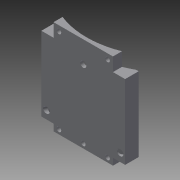
# Autodesk Inventor part: gauntlet mount
Saved by Autodesk Inventor 2014 SP1 (Build 180222100, 222)
## iProperties
Created: 2014-07-12
Part Number: gauntlet mount
Material: Generic
Document SubType Name: Modeling
Designer: Nick
Density: 1 g/cm^3
Appearance: Default
Author: Nick
Autodesk Inventor part; units mm, degrees
sketch "Sketch1" plane through (0, 0, 0) normal (0, 0, 1) x (1, 0, 0)
  line L0 (5, -2.4742) -> (53, -2.4742) construction
  line L1 (-26.0057, 3.6603) -> (-26.0057, -3.8397)
  arc A0 (0, 0) -> (58, 0) centre (29, 52.3167) ccw
  line L2 (60, -10) -> (-2, -10)
  line L3 (58, 0) -> (60, 0)
  line L4 (60, 0) -> (60, -10)
  line L5 (0, 0) -> (-2, 0)
  line L6 (-2, 0) -> (-2, -10)
  dimension "d0" = 48
  dimension "d1" = 7.5
  dimension "d2" = 58
  dimension "d16" = 2
  dimension "d17" = 2
  dimension "d18" = 10
  constraints: 14 end point, 4 perpendicular, 4 point on circle, 1 centre point, 1 horizontal, 1 parallel, 1 other
  measures "d0" distance of L0.start L0.end
  measures "d1" distance of L1.start L1.end
  measures "d2" distance of L5.start L3.start
  measures "d16" distance of L3.start L3.end
  measures "d17" distance of L5.start L5.end
  measures "d18" distance of L3.end L2.start
extrude "Extrusion1" add sketch "Sketch1" along normal blind 12
sketch3d "3D Sketch1"
ref_plane "Work Plane1" through (5, -2.4742, 6) normal (0.401226, 0.9159791, 0) x (-0.9159791, 0.401226, 0)
ref_plane "Work Plane2" through (53, -2.4742, 6) normal (-0.401226, 0.9159791, 0) x (-0.9159791, -0.401226, 0)
sketch "Sketch2" plane through (53, -2.4742, 6) normal (-0.401226, 0.9159791, 0) x (-0.9159791, -0.401226, 0)
  circle A0 centre (0, 0) radius 2.25
  point P0 (47.5542, -6)
  dimension "d9" = 4.5
  constraints: 1 centre point
  measures "d9" diameter of A0
extrude "Extrusion2" cut sketch "Sketch2" along normal mid plane 30
sketch "Sketch3" plane through (5, -2.4742, 6) normal (0.401226, 0.9159791, 0) x (-0.9159791, 0.401226, 0)
  circle A0 centre (0, 0) radius 2.25
  point P0 (5.5726, -6)
  dimension "d12" = 4.5
  constraints: 1 centre point
  measures "d12" diameter of A0
extrude "Extrusion3" cut sketch "Sketch3" along normal mid plane 30
thicken "Thicken1" operation add thickness 43 both sides no extend neighbours yes toward (0, 0, 1) faces at (29, -9.1667, 12)
sketch "Sketch4" plane through (-2, -10, 0) normal (0, -1, 0) x (1, 0, 0)
  line L0 (62, 0) -> (0, 0) projected
  line L1 (0, 55) -> (62, 55) projected
  circle A0 centre (31, 49) radius 2.25
  point P0 (2, 0)
  point P1 (31, 55)
  dimension "d21" = 4.5
  dimension "d22" = 49
  constraints: 1 centre point, 1 midpoint, 1 vertical alignment
  measures "d21" diameter of A0
  measures "d22" distance from line of L0 A0.centre
extrude "Extrusion4" cut sketch "Sketch4" against normal blind 15
sketch "Sketch5" plane through (0, 0, 0) normal (0, 0, -1) x (-1, 0, 0)
  line L0 (-58.7529, -10) -> (-55.044, -1.5326) projected
  line L1 (-53.8402, -10) -> (-50.9221, -3.3381) projected
  line L2 (0.7529, -10) -> (-2.956, -1.5326) projected
  line L3 (-4.1598, -10) -> (-7.0779, -3.3381) projected
  line L4 (-57.6988, -3.6449) -> (-59.063, -6.7592)
  line L5 (-59.063, -6.7592) -> (-52.2847, -9.7283)
  line L6 (-52.2847, -9.7283) -> (-50.9206, -6.614)
  line L7 (-50.9206, -6.614) -> (-57.6988, -3.6449)
  dimension "d25" = 7.4
  dimension "d26" = 3.4
  dimension "d27" = 3
  constraints: 8 end point, 3 parallel, 1 perpendicular
  measures "d25" distance of L4.end L5.end
  measures "d26" distance of L5.end L6.end
  measures "d27" distance from line of L7 L1.end
extrude "Extrusion5" cut sketch "Sketch5" against normal blind 10.5
ref_plane "Work Plane3" through (29, -10, 0) normal (1, 0, 0) x (0, 0, -1)
mirror "Mirror1" about plane through (29, -10, 0) normal (1, 0, 0) of "Extrusion5"
sketch "Sketch6" plane through (-2, -10, 0) normal (0, -1, 0) x (1, 0, 0)
  line L0 (62, 0) -> (0, 0) projected
  circle A0 centre (31, -1.75) radius 1.7
  circle A1 centre (49, -1.75) radius 1.7
  circle A2 centre (13, -1.75) radius 1.7
  line L1 (9, -5) -> (53, -5)
  line L2 (53, -5) -> (53, 0)
  line L3 (53, 0) -> (9, 0)
  line L4 (9, 0) -> (9, -5)
  line L5 (0, 55) -> (62, 55) projected
  line L6 (9, 55) -> (53, 55)
  line L7 (53, 55) -> (53, 65)
  line L8 (53, 65) -> (9, 65)
  line L9 (9, 65) -> (9, 55)
  circle A3 centre (13, 61) radius 1.7
  circle A4 centre (49, 61) radius 1.7
  point P0 (2, 0)
  point P1 (31, 0)
  dimension "d30" = 3.4
  dimension "d31" = 3.4
  dimension "d32" = 3.4
  dimension "d33" = 18
  dimension "d34" = 18
  dimension "d35" = 1.75
  dimension "d36" = 5
  dimension "d37" = 4
  dimension "d38" = 4
  dimension "d41" = 10
  dimension "d42" = 3.4
  dimension "d43" = 3.4
  dimension "d44" = 6
  constraints: 16 end point, 5 centre point, 4 parallel, 3 horizontal alignment, 2 horizontal, 2 perpendicular, 2 point on line, 1 midpoint, 1 vertical alignment
  measures "d30" diameter of A0
  measures "d31" diameter of A1
  measures "d32" diameter of A2
  measures "d33" distance of A0.centre A1.centre
  measures "d34" distance of A0.centre A2.centre
  measures "d35" distance from line of L0 A2.centre
  measures "d36" distance between parallel lines of L0 L1
  measures "d37" distance from line of A1.centre L2
  measures "d38" distance from line of L4 A2.centre
  measures "d41" distance of L6.end L7.end
  measures "d42" diameter of A3
  measures "d43" diameter of A4
  measures "d44" distance from line of A3.centre L6
extrude "Extrusion6" add sketch "Sketch6" against normal up to surface round surface about axis through (29, 52.3167, 0) along (0, 0, 1) radius 59.8167 far side no
body "Solid1"
